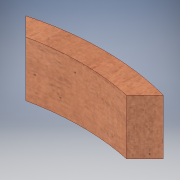
# Autodesk Inventor part: Long
Saved by Autodesk Inventor 2019 (Build 230136000, 136)
## iProperties
Created: 2019-05-01
Part Number: Long
Material: Красное дерево
Document SubType Name: Modeling
Designer: stepa
Density: 0.512 g/cm^3
Appearance: Красное дерево — натуральный — полированный
Author: stepa
Autodesk Inventor part; units mm, degrees
ref_plane "YZ Plane" through (0, 0, 0) normal (1, 0, 0) x (0, 1, 0)
ref_plane "XZ Plane" through (0, 0, 0) normal (0, 1, 0) x (-1, 0, 0)
ref_plane "XY Plane" through (0, 0, 0) normal (0, 0, 1) x (1, 0, 0)
sketch "Эскиз1" plane through (0, 0, 0) normal (0, 0, 1) x (1, 0, 0)
  line L0 (0, 0) -> (169.68, 0)
  line L1 (169.68, 0) -> (169.68, 60)
  line L2 (169.68, 60) -> (0, 60)
  line L3 (0, 60) -> (0, 0)
  dimension "d0" = 169.68
  dimension "d1" = 60
  constraints: 8 end point, 2 parallel, 1 horizontal, 1 perpendicular
  measures "d0" distance of L2.end L1.end
  measures "d1" distance of L1.end L0.end
extrude "Выдавливание1" add sketch "Эскиз1" along normal blind 30
chamfer "Фаска1" distance 30 angle 45 2 edges at (0, 30, 30) (169.68, 30, 30)
sketch "Эскиз2" plane through (0, 60, 0) normal (0, 1, 0) x (1, 0, 0)
  line L0 (0, 0) -> (169.68, 0) projected
  line L1 (84.84, 0) -> (84.84, -96.7295)
  line L2 (169.68, 0) -> (0, 0) projected
  line L3 (30, -30) -> (139.68, -30) projected
  line L4 (0, 0) -> (30, -30) projected
  arc A0 (139.68, -30) -> (30, -30) centre (84.84, -285.0513) ccw
  line L5 (139.68, -30) -> (169.68, 0) projected
  arc A1 (159.68, -10) -> (10, -10) centre (84.84, -285.0513) ccw
  point P0 (169.68, -12)
  dimension "d7" = 10
  constraints: 5 point on circle, 2 centre point, 2 end point, 2 point on line, 1 concentric, 1 midpoint, 1 perpendicular, 1 vertical, 2 other
  measures "d7" distance from line of L0 A1.end
extrude "Выдавливание2" cut sketch "Эскиз2" against normal blind 60 contours L0 A1 L4 | L0 L5 A1 | A0 L3 L1 | L1 L3 A0
